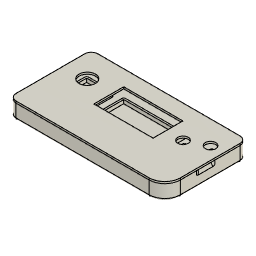
Game Console (Autodesk Fusion 360 design; units mm, degrees)
Autodesk Fusion 360 part; units mm, degrees
sketch "Skizze4" plane through (0, 0, 0) normal (0, 0, 1) x (1, 0, 0) in component "Box"
  line L0 (5, 0) -> (150, 0)
  line L1 (165, 15) -> (165, 80)
  line L2 (160, 85) -> (5, 85)
  line L3 (0, 80) -> (0, 5)
  arc A0 (5, 85) -> (0, 80) centre (5, 80) ccw
  arc A1 (165, 80) -> (160, 85) centre (160, 80) ccw
  arc A2 (0, 5) -> (5, 0) centre (5, 5) ccw
  arc A3 (150, 0) -> (165, 15) centre (150, 15) ccw
  line L4 (50.3, 19.6) -> (114.7, 19.6)
  line L5 (114.7, 19.6) -> (114.7, 70)
  line L6 (114.7, 70) -> (50.3, 70)
  line L7 (50.3, 70) -> (50.3, 19.6)
  line L8 (10, 42.6) -> (35.9, 42.6)
  line L9 (35.9, 42.6) -> (35.9, 70)
  line L10 (35.9, 70) -> (10, 70)
  line L11 (10, 70) -> (10, 42.6)
  line L12 (146.1, 49.6) -> (160, 49.6)
  line L13 (160, 49.6) -> (160, 70)
  line L14 (160, 70) -> (146.1, 70)
  line L15 (146.1, 70) -> (146.1, 49.6)
  line L16 (126.1, 39.6) -> (140, 39.6)
  line L17 (140, 39.6) -> (140, 60)
  line L18 (140, 60) -> (126.1, 60)
  line L19 (126.1, 60) -> (126.1, 39.6)
  line L20 (-2, 80) -> (-2, 5)
  arc A4 (-2, 5) -> (5, -2) centre (5, 5) ccw
  line L21 (5, -2) -> (150, -2)
  arc A5 (150, -2) -> (167, 15) centre (150, 15) ccw
  line L22 (167, 15) -> (167, 80)
  arc A6 (167, 80) -> (160, 87) centre (160, 80) ccw
  line L23 (160, 87) -> (5, 87)
  arc A7 (5, 87) -> (-2, 80) centre (5, 80) ccw
  line L24 (8, 40.6) -> (37.9, 40.6)
  line L25 (37.9, 40.6) -> (37.9, 72)
  line L26 (37.9, 72) -> (8, 72)
  line L27 (8, 72) -> (8, 40.6)
  line L28 (48.3, 17.6) -> (116.7, 17.6)
  line L29 (116.7, 17.6) -> (116.7, 72)
  line L30 (116.7, 72) -> (48.3, 72)
  line L31 (48.3, 72) -> (48.3, 17.6)
  line L32 (124.1, 37.6) -> (142, 37.6)
  line L33 (142, 37.6) -> (142, 62)
  line L34 (142, 62) -> (124.1, 62)
  line L35 (124.1, 62) -> (124.1, 37.6)
  line L36 (162, 47.6) -> (162, 72)
  line L37 (162, 72) -> (144.1, 72)
  line L38 (144.1, 72) -> (144.1, 47.6)
  line L39 (144.1, 47.6) -> (162, 47.6)
  point P0 (165, 0)
  point P1 (0, 85)
  dimension "d3" = 165
  dimension "d4" = 85
  dimension "d5" = 5
  dimension "d6" = 5
  dimension "d7" = 5
  dimension "d8" = 15
  dimension "d10" = 64.4
  dimension "d11" = 50.4
  dimension "d19" = 25.9
  dimension "d20" = 27.4
  dimension "d21" = 13.9
  dimension "d22" = 20.4
  dimension "d23" = 13.9
  dimension "d24" = 20.4
  dimension "d27" = 2
  dimension "d29" = 2
  dimension "d30" = 2
  dimension "d31" = 2
  dimension "d32" = 2
  constraint horizontal L0
  constraint vertical L1
  constraint horizontal L2
  constraint vertical L3
  constraint coincident P1 L2
  constraint coincident P1 L3
  constraint tangent L2 A0
  constraint tangent L3 A0
  constraint tangent L1 A1
  constraint tangent L2 A1
  constraint coincident origin L0
  constraint coincident origin L3
  constraint tangent L0 A2
  constraint tangent L3 A2
  constraint coincident P0 L0
  constraint coincident P0 L1
  constraint tangent L0 A3
  constraint tangent L1 A3
  constraint horizontal L4
  constraint vertical L5
  constraint horizontal L6
  constraint vertical L7
  constraint horizontal L8
  constraint vertical L9
  constraint horizontal L10
  constraint vertical L11
  constraint horizontal L12
  constraint vertical L13
  constraint horizontal L14
  constraint vertical L15
  constraint horizontal L16
  constraint vertical L17
  constraint horizontal L18
  constraint vertical L19
  measures "d3" distance of origin P0
  measures "d4" distance of origin P1
  measures "d5" radius of A0
  measures "d6" radius of A1
  measures "d7" radius of A2
  measures "d8" radius of A3
  measures "d10" distance of L4.start L4.end
  measures "d11" distance of L4.start L6.end
  measures "d19" distance of L8.start L8.end
  measures "d20" distance of L8.start L10.end
  measures "d21" distance of L12.start L12.end
  measures "d22" distance of L12.start L14.end
  measures "d23" distance of L16.start L16.end
  measures "d24" distance of L16.start L18.end
extrude "Extrusion1" add sketch "Skizze4" along normal blind 2 contours L0 L1 L2 L3 A0 A1 A2 A3 | L4 L5 L6 L7 | L8 L9 L10 L11 | L12 L13 L14 L15 | L16 L17 L18 L19 | L20 A4 L21 A5 L22 A6 L23 A7 | L24 L25 L26 L27 | L28 L29 L30 L31 | L32 L33 L34 L35 | L36 L37 L38 L39 makes body 1 in component "Box"
extrude "Extrusion2" add sketch "Skizze4" along normal blind 6 separate body contours L24 L25 L26 L27 | L28 L29 L30 L31 | L32 L33 L34 L35 | L36 L37 L38 L39 makes body 2 at (71.7667, 18.2667, 0) makes body 3 at (141.3333, 46.4, 0) makes body 4 at (37.2333, 60.8667, 0) makes body 5 at (161.3333, 56.4, 0) in component "Box"
extrude "Extrusion3" add sketch "Skizze4" along normal blind 16 separate body contours L20 A4 L21 A5 L22 A6 L23 A7 makes body 6 in component "Box"
combine "Kombinieren1" operation add target body 1 tool bodies 6 in component "Box"
fillet "Abrundung1" radius 2 8 edges at (167, 47.5, 0) (164.9497, 84.9497, 0) (82.5, 87, 0) (0.0503, 84.9497, 0) (-2, 42.5, 0) (0.0503, 0.0503, 0) (77.5, -2, 0) (162.0208, 2.9792, 0) on bodies 1 in component "Box"
sketch "Skizze1" plane through (0, 0, 16) normal (0, 0, 1) x (-1, 0, 0) in component "Deckel"
  arc A0 (-150, 0) -> (-165, -15) centre (-150, -15) ccw
  line L0 (-150, 0) -> (-5, 0)
  arc A1 (0, -5) -> (-5, 0) centre (-5, -5) ccw
  line L1 (0, -5) -> (0, -80)
  arc A2 (-5, -85) -> (0, -80) centre (-5, -80) ccw
  line L2 (-5, -85) -> (-160, -85)
  arc A3 (-165, -80) -> (-160, -85) centre (-160, -80) ccw
  line L3 (-165, -80) -> (-165, -15)
  arc A4 (-5, -87) -> (2, -80) centre (-5, -80) ccw
  line L4 (2, -80) -> (2, -5)
  arc A5 (2, -5) -> (-5, 2) centre (-5, -5) ccw
  line L5 (-5, 2) -> (-150, 2)
  arc A6 (-150, 2) -> (-167, -15) centre (-150, -15) ccw
  line L6 (-167, -15) -> (-167, -80)
  arc A7 (-167, -80) -> (-160, -87) centre (-160, -80) ccw
  line L7 (-160, -87) -> (-5, -87)
  arc A8 (-164.7, -80) -> (-160, -84.7) centre (-160, -80) ccw
  line L8 (-5, -84.7) -> (-160, -84.7)
  arc A9 (-5, -84.7) -> (-0.3, -80) centre (-5, -80) ccw
  line L9 (-0.3, -5) -> (-0.3, -80)
  arc A10 (-0.3, -5) -> (-5, -0.3) centre (-5, -5) ccw
  line L10 (-150, -0.3) -> (-5, -0.3)
  arc A11 (-150, -0.3) -> (-164.7, -15) centre (-150, -15) ccw
  line L11 (-164.7, -80) -> (-164.7, -15)
  arc A12 (-163.7, -80) -> (-160, -83.7) centre (-160, -80) ccw
  line L12 (-5, -83.7) -> (-160, -83.7)
  arc A13 (-5, -83.7) -> (-1.3, -80) centre (-5, -80) ccw
  line L13 (-1.3, -5) -> (-1.3, -80)
  arc A14 (-1.3, -5) -> (-5, -1.3) centre (-5, -5) ccw
  line L14 (-150, -1.3) -> (-5, -1.3)
  arc A15 (-150, -1.3) -> (-163.7, -15) centre (-150, -15) ccw
  line L15 (-163.7, -80) -> (-163.7, -15)
  dimension "d41" = 0.3
  dimension "d42" = 1.3
extrude "Extrusion1'" add sketch "Skizze1" along normal blind 2 separate body contours A0 L0 A1 L1 A2 L2 A3 L3 | A4 L4 A5 L5 A6 L6 A7 L7 | A8 L8 A9 L9 A10 L10 A11 L11 | A12 L12 A13 L13 A14 L14 A15 L15 makes body 7 in component "Deckel"
extrude "Extrusion2'" add sketch "Skizze1" against normal blind 2 contours A8 L8 A9 L9 A10 L10 A11 L11 bodies 7 in component "Deckel"
fillet "Abrundung2" radius 2 1 edges at (37.9, 40.6, 3) on bodies 4 in component "Box"
fillet "Abrundung3" radius 2 1 edges at (8, 40.6, 3) on bodies 4 in component "Box"
fillet "Abrundung4" radius 2 14 edges at (48.3, 72, 3) (48.3, 17.6, 3) (116.7, 72, 3) (116.7, 17.6, 3) (124.1, 62, 3) (142, 62, 3) (124.1, 37.6, 3) (142, 37.6, 3) (8, 72, 3) (37.9, 72, 3) (144.1, 47.6, 3) (162, 47.6, 3) (162, 72, 3) (144.1, 72, 3) on bodies 2 3 4 5 in component "Box"
sketch "Skizze2" plane through (0, 0, 0) normal (0, 1, 0) x (1, 0, 0) in component "Box"
  line L0 (0, -16) -> (0, -14)
  arc A0 (0, -16) -> (0, -14) centre (-1.118, -15) ccw
  line L1 (-2, -16) -> (-1, -16)
  line L2 (-1, -16) -> (-1, -11)
  line L3 (-1, -11) -> (-2, -11)
  line L4 (-2, -11) -> (-2, -16)
  arc A1 (-1, -16) -> (-2, -11) centre (-14, -16) ccw
  point P0 (-2, -16)
  point P1 (0, -16)
  dimension "d56" = 2
  dimension "d57" = 1.5
  dimension "d58" = 1
  dimension "d59" = 5
  constraint coincident P1 L0.start
  constraint vertical L0
  constraint horizontal L1
  constraint vertical L2
  constraint horizontal L3
  constraint vertical L4
  constraint coincident P0 L1.start
  constraint tangent L2 A1
  measures "d56" distance of P1 L0.end
  measures "d57" radius of A0
  measures "d58" distance of L2.end L3.end
  measures "d59" distance of P0 L3.end
move_body "Verschieben1" bodies 7 to x (1, 0, 0) y (0, 1, 0) z (0, 0, 1) at (0, -42.5, 0) in component "Deckel"
combine "Kombinieren3" operation add target body 1 tool bodies 2 3 4 5 in component "Box"
move_body "Verschieben1'" bodies 1 to x (1, 0, 0) y (0, 1, 0) z (0, 0, 1) at (0, -42.5, 0) in component "Box"
extrude "Extrusion4" add sketch "Skizze2" along normal mid plane 20 contours L0 A0 bodies 1 in component "Box"
extrude "Extrusion5" cut sketch "Skizze2" along normal mid plane 20 contours L1 L4 A1 bodies 1 in component "Box"
fillet "Abrundung5" radius 5 2 edges at (-1.2525, 10, 13.4505) (-1.2525, -10, 13.4505) on bodies 1 in component "Box"
move_body "Verschieben2" bodies 1 to x (1, 0, 0) y (0, 1, 0) z (0, 0, 1) at (-82.5, 0, 0) in component "Box"
mirror "Spiegeln1" about plane through (0, 0, 0) normal (1, 0, 0) of 3 faces at (-83.6692, 7.6409, 14.0795) (-83.5339, -2.3333, 15.0618) (-83.6692, -7.6409, 14.0795) on bodies 1 in component "Box"
move_body "Verschieben2'" bodies 7 to x (1, 0, 0) y (0, 1, 0) z (0, 0, 1) at (0, -42.5, 0) in component "Deckel"
combine "Kombinieren1'" operation cut target body 7 tool bodies 1 body 1 seen with x (1, 0, 0) y (0, 1, 0) z (0, 0, 1) at (82.5, -42.5, 0) keep tools in component "Deckel"
combine "Kombinieren4" operation cut target body 1 tool bodies 7 body 7 seen with x (1, 0, 0) y (0, 1, 0) z (0, 0, 1) at (-82.5, 42.5, 0) keep tools in component "Box"
extrude "Extrusion3'" cut 1 faces at (0.3174, -52.5, 15.099) along direction (0, -1, 0) blind 1 on bodies 7 bodies 7 in component "Deckel"
extrude "Extrusion4'" cut 1 faces at (0.3174, -32.5, 15.099) along direction (0, 1, 0) blind 1 on bodies 7 bodies 7 in component "Deckel"
move_body "Verschieben3" bodies 7 to x (1, 0, 0) y (0, 1, 0) z (0, 0, 1) at (0, 42.5, 0) in component "Deckel"
move_body "Verschieben4" bodies 7 to x (1, 0, 0) y (0, 1, 0) z (0, 0, 1) at (-82.5, 0, 0) in component "Deckel"
mirror "Spiegeln1'" about plane through (0, 0, 0) normal (1, 0, 0) of 3 faces at (-82.136, 3.6667, 15.2315) (-82.1826, -11, 15.099) (-82.1826, 11, 15.099) on bodies 7 in component "Deckel"
mirror "Spiegeln2" about plane through (0, 0, 0) normal (1, 0, 0) of 3 faces at (-82.2042, 3.3333, 15.501) (-82.2837, -10, 15) (-82.4555, 10, 14.7244) on bodies 1 in component "Box"
sketch "Skizze2 (2)" plane through (0, 0, 6) normal (0, 0, 1) x (-1, 0, 0) in component "Deckel"
  arc A0 (44.6, -27.5) -> (46.6, -29.5) centre (46.6, -27.5) ccw
  line L0 (46.6, -29.5) -> (72.5, -29.5)
  arc A1 (72.5, -29.5) -> (74.5, -27.5) centre (72.5, -27.5) ccw
  line L1 (74.5, -27.5) -> (74.5, -0.1)
  arc A2 (74.5, -0.1) -> (72.5, 1.9) centre (72.5, -0.1) ccw
  line L2 (72.5, 1.9) -> (46.6, 1.9)
  arc A3 (46.6, 1.9) -> (44.6, -0.1) centre (46.6, -0.1) ccw
  line L3 (44.6, -0.1) -> (44.6, -27.5)
  line L4 (72.5, -0.1) -> (72.5, -27.5)
  line L5 (72.5, -27.5) -> (46.6, -27.5)
  line L6 (46.6, -27.5) -> (46.6, -0.1)
  line L7 (46.6, -0.1) -> (72.5, -0.1)
  line L8 (32.2, 22.9) -> (32.2, -27.5)
  line L9 (32.2, -27.5) -> (-32.2, -27.5)
  line L10 (-32.2, -27.5) -> (-32.2, 22.9)
  line L11 (-32.2, 22.9) -> (32.2, 22.9)
  arc A4 (-32.2, 24.9) -> (-34.2, 22.9) centre (-32.2, 22.9) ccw
  line L12 (-34.2, 22.9) -> (-34.2, -27.5)
  arc A5 (-34.2, -27.5) -> (-32.2, -29.5) centre (-32.2, -27.5) ccw
  line L13 (-32.2, -29.5) -> (32.2, -29.5)
  arc A6 (32.2, -29.5) -> (34.2, -27.5) centre (32.2, -27.5) ccw
  line L14 (34.2, -27.5) -> (34.2, 22.9)
  arc A7 (34.2, 22.9) -> (32.2, 24.9) centre (32.2, 22.9) ccw
  line L15 (32.2, 24.9) -> (-32.2, 24.9)
  line L16 (-43.6, 2.9) -> (-43.6, -17.5)
  line L17 (-43.6, -17.5) -> (-57.5, -17.5)
  line L18 (-57.5, -17.5) -> (-57.5, 2.9)
  line L19 (-57.5, 2.9) -> (-43.6, 2.9)
  arc A8 (-57.5, 4.9) -> (-59.5, 2.9) centre (-57.5, 2.9) ccw
  line L20 (-59.5, 2.9) -> (-59.5, -17.5)
  arc A9 (-59.5, -17.5) -> (-57.5, -19.5) centre (-57.5, -17.5) ccw
  line L21 (-57.5, -19.5) -> (-43.6, -19.5)
  arc A10 (-43.6, -19.5) -> (-41.6, -17.5) centre (-43.6, -17.5) ccw
  line L22 (-41.6, -17.5) -> (-41.6, 2.9)
  arc A11 (-41.6, 2.9) -> (-43.6, 4.9) centre (-43.6, 2.9) ccw
  line L23 (-43.6, 4.9) -> (-57.5, 4.9)
  line L24 (-63.6, -7.1) -> (-63.6, -27.5)
  line L25 (-63.6, -27.5) -> (-77.5, -27.5)
  line L26 (-77.5, -27.5) -> (-77.5, -7.1)
  line L27 (-77.5, -7.1) -> (-63.6, -7.1)
  arc A12 (-63.6, -29.5) -> (-61.6, -27.5) centre (-63.6, -27.5) ccw
  line L28 (-61.6, -27.5) -> (-61.6, -7.1)
  arc A13 (-61.6, -7.1) -> (-63.6, -5.1) centre (-63.6, -7.1) ccw
  line L29 (-63.6, -5.1) -> (-77.5, -5.1)
  arc A14 (-77.5, -5.1) -> (-79.5, -7.1) centre (-77.5, -7.1) ccw
  line L30 (-79.5, -7.1) -> (-79.5, -27.5)
  arc A15 (-79.5, -27.5) -> (-77.5, -29.5) centre (-77.5, -27.5) ccw
  line L31 (-77.5, -29.5) -> (-63.6, -29.5)
  line L32 (44.6, -0.1) -> (44.6, -27.5)
  line L33 (32.2, -27.5) -> (-32.2, -27.5)
  line L34 (-32.2, -27.5) -> (-32.2, 4.9)
  line L35 (-32.2, 4.9) -> (32.2, 4.9)
  line L36 (32.2, 4.9) -> (32.2, -27.5)
  circle A16 centre (-50.55, -9.3353) radius 5.75
  circle A17 centre (-70.55, -19.3139) radius 5.75
  circle A18 centre (59.55, -15.2085) radius 8.95
  dimension "d78" = 32.4
  dimension "d80" = 11.5
  dimension "d81" = 11.5
  dimension "d88" = 17.9
  constraint horizontal L33
  constraint vertical L34
  constraint horizontal L35
  constraint vertical L36
  constraint coincident L10 L34.end
  constraint coincident L8.end L9.start
  measures "d78" distance of L8.end L35.end
  measures "d80" diameter of A16
  measures "d81" diameter of A17
  measures "d88" diameter of A18
extrude "Extrusion5'" cut sketch "Skizze2 (2)" along normal blind 20 contours L8 L10 L11 L35 | L8 L9 L10 L33 L34 L35 L36 bodies 7 in component "Deckel"
move_face "Flächen versetzen1" offset 18 1 faces at (10.7333, -22.9, 16.6667) on bodies 7 in component "Deckel"
extrude "Extrusion6" cut sketch "Skizze2 (2)" along normal blind 12 contours A16 bodies 7 in component "Deckel"
extrude "Extrusion7" cut sketch "Skizze2 (2)" along normal blind 11 contours A17 bodies 7 in component "Deckel"
extrude "Extrusion8" cut sketch "Skizze2 (2)" along normal blind 12 contours A17 bodies 7 in component "Deckel"
extrude "Extrusion9" cut sketch "Skizze2 (2)" along normal blind 20 contours A18 bodies 7 in component "Deckel"
sketch "Skizze3" plane through (-84.5, 0, 0) normal (-1, 0, 0) x (0, -1, 0) in component "Box"
  line L0 (-37.5, 16) -> (37.5, 16)
  line L1 (37.5, 16) -> (37.5, 18)
  line L2 (37.5, 18) -> (-37.5, 18)
  line L3 (-37.5, 18) -> (-37.5, 16)
  line L4 (21.6, 6.4) -> (30, 6.4)
  line L5 (30, 6.4) -> (30, 2)
  line L6 (30, 2) -> (21.6, 2)
  line L7 (21.6, 2) -> (21.6, 6.4)
  dimension "d91" = 8.4
  dimension "d92" = 4.4
  constraint horizontal L4
  constraint vertical L5
  constraint horizontal L6
  constraint vertical L7
  measures "d91" distance of L5.end L6.end
  measures "d92" distance of L4.start L6.end
extrude "Extrusion6'" cut sketch "Skizze3" against normal blind 5 contours L4 L5 L6 L7 bodies 1 in component "Box"
combine "Kombinieren2" [suppressed] in component "Box"
extrude "Extrusion1''" [suppressed] in component "Box"
extrude "Extrusion2''" [suppressed] in component "Box"
extrude "Extrusion3''" [suppressed] in component "Box"
component "Box" placed x (1, 0, 0) y (0, 1, 0) z (0, 0, 1) at (0, 0, 0)
component "Deckel" placed x (1, 0, 0) y (0, 1, 0) z (0, 0, 1) at (0, 0, 0)
